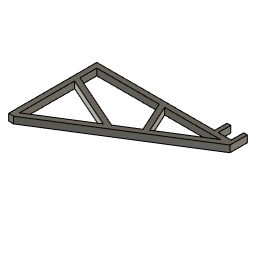
non triangle supports v3 (Autodesk Fusion 360 design; units mm, degrees)
Autodesk Fusion 360 part; units mm, degrees
sketch "Sketch1" plane through (0, 0, 0) normal (0, 0, 1) x (1, 0, 0)
  line L0 (0, 0) -> (7.62, 0)
  line L1 (7.62, 0) -> (7.62, 134.62)
  line L2 (7.62, 134.62) -> (0, 134.62)
  line L3 (0, 134.62) -> (0, 0)
  line L4 (7.62, 134.62) -> (210.82, 134.62)
  line L5 (210.82, 134.62) -> (210.82, 127)
  line L6 (210.82, 127) -> (7.62, 127)
  line L7 (7.62, 127) -> (7.62, 134.62)
  line L8 (210.82, 127) -> (7.62, 0)
  line L9 (7.62, 0) -> (3.5814, 6.4617)
  line L10 (3.5814, 6.4617) -> (206.7814, 133.4617)
  line L11 (206.7814, 133.4617) -> (210.82, 127)
  line L12 (210.82, 134.62) -> (205.105, 134.62)
  line L13 (205.105, 134.62) -> (205.105, 153.67)
  line L14 (205.105, 153.67) -> (210.82, 153.67)
  line L15 (210.82, 153.67) -> (210.82, 134.62)
  line L16 (185.4311, 134.62) -> (179.7161, 134.62)
  line L17 (179.7161, 134.62) -> (179.7161, 153.67)
  line L18 (179.7161, 153.67) -> (185.4311, 153.67)
  line L19 (185.4311, 153.67) -> (185.4311, 134.62)
  line L20 (0, 96.52) -> (91.44, 55.88)
  line L21 (91.44, 55.88) -> (94.5348, 62.8432)
  line L22 (94.5348, 62.8432) -> (3.0948, 103.4832)
  line L23 (3.0948, 103.4832) -> (0, 96.52)
  line L24 (132.08, 81.28) -> (109.22, 131.3392)
  line L25 (109.22, 131.3392) -> (102.2885, 128.1739)
  line L26 (102.2885, 128.1739) -> (125.1485, 78.1147)
  line L27 (125.1485, 78.1147) -> (132.08, 81.28)
  dimension "d1" = 134.62
  dimension "d2" = 7.62
  dimension "d3" = 203.2
  dimension "d4" = 7.62
  dimension "d5" = 19.05
  dimension "d6" = 5.715
  dimension "d7" = 5.715
  dimension "d8" = 19.05
  dimension "d9" = 7.62
  dimension "d10" = 7.62
  constraint horizontal L0
  constraint vertical L1
  constraint horizontal L2
  constraint vertical L3
  constraint coincident L0.start L3.end
  constraint horizontal L4
  constraint vertical L5
  constraint horizontal L6
  constraint vertical L7
  constraint perpendicular L8 L9
  constraint parallel L8 L10
  constraint parallel L9 L11
  constraint horizontal L12
  constraint vertical L13
  constraint horizontal L14
  constraint vertical L15
  constraint horizontal L16
  constraint vertical L17
  constraint horizontal L18
  constraint vertical L19
  constraint coincident L4 L16.start
  constraint perpendicular L20 L21
  constraint parallel L20 L22
  constraint parallel L21 L23
  constraint coincident L3 L20.start
  constraint perpendicular L24 L25
  constraint parallel L24 L26
  constraint parallel L25 L27
  measures "d1" distance of L0.start L2.end
  measures "d2" distance of L0.start L0.end
  measures "d3" distance of L1.end L4.end
  measures "d4" distance of L5.end L10.end
  measures "d5" distance of L4.end L14.end
  measures "d6" distance of L4.end L12.end
  measures "d7" distance of L16.start L16.end
  measures "d8" distance of L16.start L18.end
  measures "d9" distance of L20.start L22.end
  measures "d10" distance of L24.start L26.end
extrude "Extrude1" add sketch "Sketch1" along normal blind 10.16 contours L0 L1 L3 L9 L10 L20 | L1 L9 L10 | L1 L6 L8 L10 L20 L21 L22 L24 L26 L27 | L1 L20 L22 L23 | L1 L2 L3 L7 L22 L23 | L1 L4 L5 L6 L7 L10 L11 L12 L16 L24 L25 L26 | L6 L10 L11 | L1 L10 L20 L22 | L10 L20 L21 L22 | L4 L12 L13 L14 L15 | L6 L10 L24 L26 | L6 L24 L25 L26 | L10 L24 L26 L27 | L4 L16 L17 L18 L19
